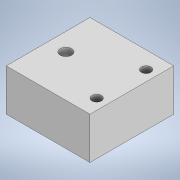
# Autodesk Inventor part: SpoutHolder
Saved by Autodesk Inventor 2020.4 (Build 244396010, 396A)
## iProperties
Created: 2022-09-17
Part Number: SpoutHolder
Material: Generic
Document SubType Name: Modeling
Designer: YUSTE
Density: 1 g/cm^3
Appearance: Default
Author: YUSTE
Autodesk Inventor part; units mm, degrees
ref_plane "YZ Plane" through (0, 0, 0) normal (1, 0, 0) x (0, 1, 0)
ref_plane "XZ Plane" through (0, 0, 0) normal (0, 1, 0) x (-1, 0, 0)
ref_plane "XY Plane" through (0, 0, 0) normal (0, 0, 1) x (1, 0, 0)
sketch "Sketch1" plane through (0, 0, 0) normal (0, 1, 0) x (-1, 0, 0)
  line L0 (0, 0) -> (0, 50.8)
  line L1 (0, 50.8) -> (50.8, 50.8)
  line L2 (50.8, 50.8) -> (50.8, 0)
  line L3 (50.8, 0) -> (0, 0)
  circle A0 centre (6.35, 40.4012) radius 2.8956
  circle A1 centre (6.35, 10.4013) radius 2.8956
  circle A2 centre (39.9999, 25.4) radius 3.4925
  dimension "d0" = 50.8
  dimension "d1" = 50.8
  dimension "d2" = 5.7912
  dimension "d3" = 5.7912
  dimension "d4" = 29.9999
  dimension "d5" = 10.4013
  dimension "d6" = 6.35
  dimension "d7" = 6.35
  dimension "d8" = 6.985
  dimension "d9" = 39.9999
  dimension "d10" = 25.4
  constraints: 8 end point, 3 centre point, 2 parallel, 1 perpendicular, 1 vertical
  measures "d0" distance of L0.start L0.end
  measures "d1" distance of L0.end L1.end
  measures "d2" diameter of A0
  measures "d3" diameter of A1
  measures "d4" distance of A1.centre A0.centre
  measures "d5" distance from line of L3 A1.centre
  measures "d6" distance from line of L0 A0.centre
  measures "d7" distance from line of L0 A1.centre
  measures "d8" diameter of A2
  measures "d9" distance from line of L0 A2.centre
  measures "d10" distance from line of L1 A2.centre
extrude "Extrusion1" add sketch "Sketch1" along normal blind 25.4
body "Solid1"
